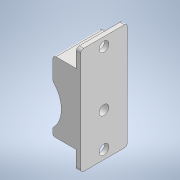
# Autodesk Inventor part: Motor Cleat
Saved by Autodesk Inventor 2022 (Build 260153000, 153)
## iProperties
Created: 2022-09-25
Part Number: Motor Cleat
Material: Generic
Document SubType Name: Modeling
Designer: matt
Density: 1 g/cm^3
Appearance: Default
Author: matt
Autodesk Inventor part; units mm, degrees
ref_plane "YZ Plane" through (0, 0, 0) normal (1, 0, 0) x (0, 1, 0)
ref_plane "XZ Plane" through (0, 0, 0) normal (0, 1, 0) x (-1, 0, 0)
sketch "Sketch1" plane through (0, 0, 0) normal (0, 0, 1) x (1, 0, 0)
  arc A0 (23.7707, 5.756) -> (23.9448, 31.7775) centre (10.4963, 18.8562) ccw
  line L0 (42.91, 38.9085) -> (39.91, 38.8609)
  line L1 (42.91, -0.4) -> (39.91, -0.4)
  line L2 (23.1942, 4.3512) -> (23.1942, 1.6)
  line L3 (39.91, 60.7501) -> (42.91, 60.7501)
  line L4 (42.91, 60.7501) -> (42.91, -23.2499)
  line L5 (42.91, -23.2499) -> (39.91, -23.2499)
  line L6 (39.91, -23.2499) -> (39.91, -0.4)
  line L7 (39.91, 38.8609) -> (39.91, 60.7501)
  line L8 (39.91, -23.2499) -> (39.91, -0.4)
  line L9 (39.91, -0.4) -> (39.91, 60.7501)
  arc A1 (23.1942, 1.6) -> (25.1942, -0.4) centre (25.1942, 1.6) ccw
  arc A2 (23.387, 33.1631) -> (23.9448, 31.7775) centre (25.387, 33.1631) ccw
  arc A3 (23.7707, 5.756) -> (23.1942, 4.3512) centre (25.1942, 4.3512) ccw
  line L10 (39.91, 38.8609) -> (25.3553, 38.63)
  line L11 (39.91, -0.4) -> (25.1942, -0.4)
  line L12 (40.0772, 38.3635) -> (25.3632, 38.13)
  line L13 (23.887, 36.6302) -> (23.887, 33.1631)
  arc A4 (23.887, 33.1631) -> (24.3054, 32.1239) centre (25.387, 33.1631) ccw
  arc A5 (24.1266, 5.4048) -> (24.3054, 32.1239) centre (10.4963, 18.8562) ccw
  arc A6 (24.1266, 5.4048) -> (23.6942, 4.3512) centre (25.1942, 4.3512) ccw
  line L14 (23.6942, 4.3512) -> (23.6942, 1.6)
  arc A7 (23.6942, 1.6) -> (25.1942, 0.1) centre (25.1942, 1.6) ccw
  line L15 (25.1942, 0.1) -> (39.91, 0.1)
  line L16 (39.91, 48.2501) -> (25.887, 48.2501)
  line L17 (23.887, 36.6302) -> (23.887, 46.2501)
  arc A8 (25.887, 48.2501) -> (23.887, 46.2501) centre (25.887, 46.2501) ccw
  point P0 (0, 0)
  point P1 (23.1942, 5.1965)
  point P2 (23.387, 32.334)
  point P3 (36.735, -12.4)
  point P4 (39.91, -12.3999)
  point P5 (39.91, 38.3609)
  dimension "d0" = 3
  dimension "d38" = 2
  constraints: 36 end point, 20 point on circle, 9 centre point, 8 tangent, 5 perpendicular, 5 point on line, 3 parallel, 2 vertical, 1 equal radius, 1 horizontal, 8 other
  measures "d0" distance of L4.end L5.end
  measures "d38" radius of A8
ref_plane "Work Plane1" through (39.91, -23.2499, 0) normal (-1, 0, 0) x (0, 0, 1)
extrude "Extrusion3" add sketch "Sketch1" along normal blind 32
sketch "Sketch4" plane through (42.91, -23.2499, 0) normal (1, 0, 0) x (0, 0, -1)
  circle A0 centre (-16, 78) radius 3.35
  circle A1 centre (-16, 16.85) radius 3.35
  line L0 (0, 0) -> (0, 84) projected
  line L1 (-32, 0) -> (-32, 84) projected
  line L2 (-32, 23.3499) -> (-32, 0) projected
  line L3 (-32, 10.85) -> (0, 10.85)
  line L4 (0, 23.3499) -> (0, 0) projected
  line L5 (0, 84) -> (-32, 84) projected
  line L6 (0, 0) -> (-32, 0) projected
  line L7 (-32, 0) -> (0, 0)
  line L8 (-16, 84) -> (-16, 10.85) construction
  circle A2 centre (-16, 40.3809) radius 3.3
  point P0 (0, 23.2499)
  dimension "d23" = 6.7
  dimension "d26" = 32
  dimension "d31" = 73.15
  dimension "d33" = 6
  dimension "d34" = 6
  dimension "d39" = 6.6
  constraints: 6 end point, 4 point on line, 3 centre point, 2 midpoint, 1 collinear, 1 equal radius, 1 perpendicular
  measures "d23" diameter of A0
  measures "d26" distance between parallel lines of L0 L1
  measures "d31" distance between parallel lines of L3 L5
  measures "d33" distance from line of L5 A0.centre
  measures "d34" distance from line of L3 A1.centre
  measures "d39" diameter of A2
extrude "Extrusion4" cut sketch "Sketch4" against normal blind 32 contours A0 | A1 | L6 L1 L3 L0 | A2
fillet "Fillet3" radius 2 4 edges at (41.41, 60.7501, 32) (41.41, 60.7501, 0) (41.41, -12.3999, 0) (41.41, -12.3999, 32)
body "Solid2"
